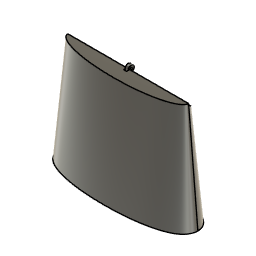
handsupport_final (Autodesk Fusion 360 design; units mm, degrees)
Autodesk Fusion 360 part; units mm, degrees
sketch "Sketch1" plane through (0, 0, 0) normal (0, 0, 1) x (1, 0, 0)
  ellipse E0 centre (0, 0) end of major axis (-60, 0) minor radius 15
  line L0 (60, 0) -> (-60, 0) construction
  line L1 (0, 15) -> (0, -15) construction
  dimension "d1" = 120
  dimension "d2" = 30
  constraint coincident E0 L0.start
  constraint coincident E0 L0.end
  constraint coincident E0 L1.start
  constraint coincident E0 L1.end
  constraint coincident E0.centre origin
  constraint horizontal L0
  measures "d1" distance of E0
extrude "Extrude1" add sketch "Sketch1" against normal blind 105 draft 5 makes body 1
sketch "Sketch2" plane through (0, 0, 0) normal (1, 0, 0) x (0, 1, 0)
  line L0 (0, 0) -> (0, -1)
  line L1 (0, -1) -> (20.025, -21.025)
  line L2 (0, -1) -> (28.3196, -1) construction
  line L3 (20.025, -21.025) -> (22, 9)
  line L4 (22, 9) -> (0, 0)
  dimension "d5" = 1
  dimension "d6" = 45
  constraint coincident L0.start L4.end
  constraint vertical L0
  constraint horizontal L2
  measures "d5" distance of L0.start L0.end
  measures "d6" angle of L1 L2
extrude "Extrude2" cut sketch "Sketch2" along normal mid plane 200 bodies 1
sketch "Sketch3" plane through (0, 0, 0) normal (0, 1, 0) x (-1, 0, 0)
  line L0 (-60, 0) -> (-60.0875, -1)
  line L1 (-60.0875, -1) -> (60.0875, -1)
  line L2 (60, 0) -> (60.0875, -1)
  line L3 (60, 0) -> (-60, 0)
  line L4 (0, 0) -> (1.5, 0)
  line L5 (1.5, 0) -> (1.5, -3)
  line L6 (1.5, -3) -> (0, -3)
  line L7 (0, -3) -> (0, 0)
  line L8 (0, 0) -> (-1.5, 0)
  line L9 (-1.5, 0) -> (-1.5, -3)
  line L10 (-1.5, -3) -> (0, -3)
  line L11 (0, -3) -> (0, 0)
  dimension "d9" = 1.5
  dimension "d10" = 3
  dimension "d11" = 1.5
  dimension "d12" = 3
  constraint horizontal L4
  constraint vertical L5
  constraint horizontal L6
  constraint vertical L7
  constraint coincident L4.start L7.end
  constraint horizontal L8
  constraint vertical L9
  constraint horizontal L10
  constraint vertical L11
  measures "d9" distance of L4.start L4.end
  measures "d10" distance of L4.start L6.end
  measures "d11" distance of L4.start L8.end
  measures "d12" distance of L4.start L6.end
extrude "Extrude3" cut sketch "Sketch3" along normal mid plane 6 contours L1 L3 L7 L8 L9 L11 | L1 L7 L9 L10 L11 | L1 L3 L4 L5 L7 L11 | L1 L5 L6 L7 L11 bodies 1
ref_plane "WorkPlane1" through (0, -0.5, -1.5) normal (1, 0, 0) x (0, 0, -1)
sketch "Sketch4" plane through (0, 0, 0) normal (1, 0, 0) x (0, 1, 0)
  circle A0 centre (1.5, 0) radius 1.25
  circle A1 centre (1.5, 0) radius 3
  dimension "d15" = 2.5
  dimension "d16" = 6
  dimension "d17" = 1.5
  constraint concentric A0 A1
  measures "d15" diameter of A0
  measures "d16" diameter of A1
  measures "d17" distance of origin A0.centre
extrude "Extrude4" add sketch "Sketch4" along normal mid plane 3 separate body makes body 2
